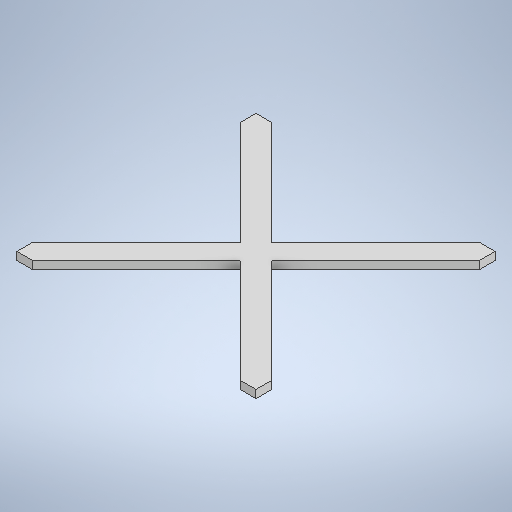
# Autodesk Inventor part: 적재부 상판
Saved by Autodesk Inventor 2025 (Build 290162000, 162)
## iProperties
Created: 2024-06-08
Part Number: 적재부 상판
Material: 일반
Document SubType Name: Modeling
Designer: goomi
Density: 1 g/cm^3
Appearance: 기본값
Author: goomi
Autodesk Inventor part; units mm, degrees
ref_plane "YZ Plane" through (0, 0, 0) normal (1, 0, 0) x (0, 1, 0)
ref_plane "XZ Plane" through (0, 0, 0) normal (0, 1, 0) x (-1, 0, 0)
ref_plane "XY Plane" through (0, 0, 0) normal (0, 0, 1) x (1, 0, 0)
sketch "스케치1" plane through (0, 0, 0) normal (0, 1, 0) x (-1, 0, 0)
  line L0 (150, 0) -> (140, 0)
  line L1 (140, 0) -> (140, -5)
  line L2 (140, -5) -> (145, -5)
  line L3 (150, -5) -> (150, 0)
  line L4 (150, 0) -> (145, 0)
  line L5 (145, -5) -> (145, -10)
  line L6 (145, -10) -> (150, -10)
  line L7 (150, -10) -> (150, 0)
  line L8 (150, -75) -> (0, -75)
  line L9 (75, 0) -> (75, -150)
  line L10 (140, -150) -> (140, -145)
  line L11 (140, -145) -> (145, -145)
  line L12 (145, -145) -> (145, -140)
  line L13 (145, -140) -> (150, -140)
  line L14 (75, -150) -> (75, 0)
  line L15 (10, 0) -> (10, -5)
  line L16 (10, -5) -> (5, -5)
  line L17 (5, -5) -> (5, -10)
  line L18 (5, -10) -> (0, -10)
  line L19 (10, -150) -> (10, -145)
  line L20 (10, -145) -> (5, -145)
  line L21 (5, -140) -> (0, -140)
  line L22 (5, -145) -> (5, -140)
  line L23 (140, 0) -> (0, -140)
  line L24 (10, -150) -> (150, -10)
  line L25 (150, -140) -> (10, 0)
  line L26 (0, -10) -> (140, -150)
  line L27 (0, 0) -> (10, 0)
  line L28 (140, 0) -> (150, 0)
  line L29 (0, -150) -> (0, -140)
  line L30 (0, -10) -> (0, 0)
  line L31 (150, -150) -> (140, -150)
  line L32 (10, -150) -> (0, -150)
  line L33 (150, 0) -> (150, -10)
  line L34 (150, -140) -> (150, -150)
  point P0 (75, -65)
  point P1 (65, -75)
  point P2 (75, -85)
  point P3 (85, -75)
  dimension "d0" = 150
  dimension "d1" = 150
  dimension "d2" = 10
  dimension "d3" = 5
  dimension "d4" = 5
  dimension "d5" = 10
  constraints: 70 end point, 17 symmetric about line, 13 parallel, 7 perpendicular, 4 horizontal
  measures "d0" distance of L31.start L29.start
  measures "d1" distance of L0.start L31.start
  measures "d2" distance of L3.start L1.end
  measures "d3" distance of L1.end L0.end
  measures "d4" distance of L6.end L5.end
  measures "d5" distance of L5.end L4.end
extrude "돌출1" add sketch "스케치1" along normal blind 5
